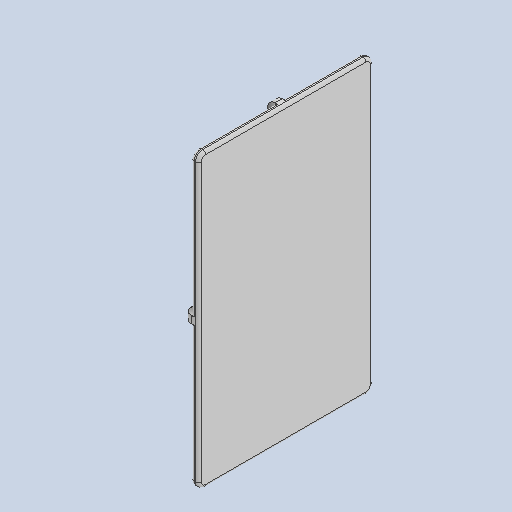
# Autodesk Inventor part: Fastener 2
Saved by Autodesk Inventor 2022 (Build 260153000, 153)
## iProperties
Created: 2023-10-19
Part Number: Fastener 2
Material: Типовые
Document SubType Name: Modeling
Designer: user
Density: 1 g/cm^3
Appearance: По умолчанию
Author: user
## iProperties of the stored document Fastener 2 horizontal_3DПЕЧАТЬ.ipt
Created: 2023-10-22
Part Number: Fastener 2 horizontal_3DПЕЧАТЬ
Material: Типовые
Document SubType Name: Modeling
Designer: user
Density: 1 g/cm^3
Appearance: По умолчанию
Author: user
Autodesk Inventor part; units mm, degrees
ref_plane "YZ Plane" through (0, 0, 0) normal (1, 0, 0) x (0, 1, 0)
ref_plane "XZ Plane" through (0, 0, 0) normal (0, 1, 0) x (-1, 0, 0)
ref_plane "РабПлоскость1" through (0, 0, 0) normal (0, 0, 1) x (1, 0, 0)
sketch "Эскиз1" plane through (0, 0, 0) normal (0, 0, 1) x (1, 0, 0)
  circle A0 centre (0, 0) radius 3
  circle A1 centre (0, 0) radius 6
  line L0 (-2.5202, -5.4451) -> (12, -12.1655)
  line L1 (-2.5202, 5.4451) -> (12, 12.1655)
  line L2 (12, -12.1655) -> (12, 12.1655)
  line L3 (-9.6, 0) -> (15.6, 0) projected
  point P0 (0, 0)
  point P1 (12, 0)
  dimension "d0" = 12
  dimension "d1" = 12
  dimension "d2" = 16
  dimension "d23" = 6
  constraints: 6 end point, 2 centre point, 2 coincident, 2 point on circle, 2 tangent, 1 equal length, 1 midpoint, 1 point on line
  measures "d0" diameter of A1
  measures "d1" distance from line of L2 A0.centre
  measures "d2" distance of L0.start L0.end
  measures "d23" diameter of A0
extrude "Выдавливание1" add sketch "Эскиз1" along normal blind 6 contours L3 A1 A0 | A0 L3 A1 | L3 L2 L0 A1 | A1 L1 L2 L3
sketch "Эскиз2" plane through (12, 12.1655, 6) normal (1, 0, 0) x (0, 0, -1)
  line L0 (-47, -42.1655) -> (53, -42.1655)
  line L1 (53, -42.1655) -> (53, 17.8345)
  line L2 (53, 17.8345) -> (-47, 17.8345)
  line L3 (-47, 17.8345) -> (-47, -42.1655)
  line L4 (6, -24.3311) -> (0, -24.3311) projected
  line L5 (3, -24.3311) -> (3, 0) construction
  line L6 (6, 0) -> (0, 0) projected
  line L7 (0, -6.7205) -> (0, -17.6106) projected
  line L8 (0, -12.1655) -> (6, -12.1655) construction
  line L9 (33, 37.8345) -> (-27, 37.8345)
  line L10 (-27, 37.8345) -> (-27, -62.1655)
  line L11 (-27, -62.1655) -> (33, -62.1655)
  line L12 (33, -62.1655) -> (33, 37.8345)
  line L13 (33, -12.1655) -> (-27, -12.1655) construction
  line L14 (3, 37.8345) -> (3, -62.1655) construction
  point P0 (3, 0)
  point P1 (0, -12.1655)
  dimension "d6" = 100
  dimension "d7" = 60
  dimension "d8" = 30
  dimension "d9" = 50
  dimension "d19" = 60
  dimension "d20" = 100
  constraints: 24 end point, 9 midpoint, 4 parallel, 3 horizontal, 2 perpendicular, 2 point on line
  measures "d6" distance between parallel lines of L1 L3
  measures "d7" distance between parallel lines of L0 L2
  measures "d8" distance between parallel lines of L2 L8
  measures "d9" distance between parallel lines of L3 L5
  measures "d19" distance of L11.end L10.end
  measures "d20" distance of L10.end L9.end
extrude "Выдавливание2" add sketch "Эскиз2" along normal blind 2.5 contours L10 L2 L12 L0 | L0 L12 L11 L10 | L10 L9 L12 L2
sketch "Эскиз3" plane through (12, 12.1655, 6) normal (-1, 0, 0) x (0, 0, 1)
  line L0 (27, -13.4155) -> (-33, -13.4155)
  line L1 (-33, -13.4155) -> (-33, -10.9155)
  line L2 (-33, -10.9155) -> (27, -10.9155)
  line L3 (27, -10.9155) -> (27, -13.4155)
  line L4 (27, -12.1655) -> (-33, -12.1655) construction
  line L5 (-1.75, 37.8345) -> (-1.75, -62.1655)
  line L6 (-4.25, -62.1655) -> (-4.25, 37.8345)
  line L7 (-6, -24.3311) -> (0, -24.3311) projected
  line L8 (-3, -24.3311) -> (-3, 0) construction
  line L9 (-6, 0) -> (0, 0) projected
  line L10 (-33, 37.8345) -> (27, 37.8345) projected
  line L11 (27, 37.8345) -> (27, -62.1655) projected
  line L12 (-33, -62.1655) -> (-33, 37.8345) projected
  line L13 (27, -62.1655) -> (-33, -62.1655) projected
  line L14 (0, -17.6106) -> (0, -6.7205) projected
  point P0 (-1.75, -13.4155)
  point P1 (-4.25, -13.4155)
  point P2 (-4.25, -10.9155)
  point P3 (-1.75, -10.9155)
  point P4 (0, -12.1655)
  point P5 (-1.75, -24.3311)
  point P6 (-4.25, -24.3311)
  point P7 (-4.25, 0)
  point P8 (-1.75, 0)
  dimension "d12" = 2.5
  dimension "d16" = 2.5
  dimension "d17" = 1.25
  constraints: 16 end point, 5 midpoint, 5 point on line, 2 collinear, 2 parallel, 1 horizontal, 1 perpendicular
  measures "d12" distance between parallel lines of L2 L0
  measures "d16" distance between parallel lines of L6 L5
  measures "d17" distance between parallel lines of L6 L8
extrude "Выдавливание3" add sketch "Эскиз3" along normal blind 2.5 contours L0 L14 L2 L3 | L0 L5 L2 L14 | L5 L7 L6 L0 | L0 L6 L2 L5 | L13 L6 L7 L5 | L0 L1 L2 L6 | L2 L6 L9 L5 | L5 L9 L6 L10
fillet "Сопряжение1" radius 2.5 4 edges at (9.5, 0, 33) (9.5, 0, -27) (9.5, 50, 3) (9.5, -50, 3)
fillet "Сопряжение2" radius 2.5 4 edges at (13.25, 50, 33) (13.25, -50, 33) (13.25, 50, -27) (13.25, -50, -27)
fillet "Сопряжение3" radius 1 20 edges at (14.5, 49.2678, 32.2678) (14.5, 0, 33) (14.5, -49.2678, 32.2678) (14.5, -50, 3) (14.5, -49.2678, -26.2678) (14.5, 0, -27) (14.5, 49.2678, -26.2678) (14.5, 50, 3) (12, 49.2678, 32.2678) (12, 24.375, 33) (12, 50, 17.375) (12, 49.2678, -26.2678) (12, 24.375, -27) (12, 50, -11.375) (12, -24.375, -27) (12, -50, -11.375) (12, -49.2678, -26.2678) (12, -49.2678, 32.2678) (12, -24.375, 33) (12, -50, 17.375)
fillet "Сопряжение4" radius 4 16 edges at (12, 6.7078, 6) (12, 12.1655, 5.125) (12, 12.1655, 0.875) (12, 6.7078, 0) (9.5, 0, 0) (12, -6.7078, 0) (12, -12.1655, 0.875) (12, -12.1655, 5.125) (12, -6.7078, 6) (9.5, 0, 6) (10.75, -1.25, 6) (10.75, 1.25, 6) (10.75, 1.25, 0) (10.75, -1.25, 0) (9.5, -11.0084, 3) (9.5, 11.0084, 3)
